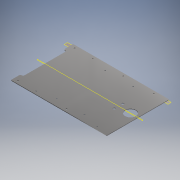
# Autodesk Inventor part: Back
Saved by Autodesk Inventor 2018 (Build 220112000, 112)
## iProperties
Created: 2017-11-12
Part Number: Back
Material: Edelstahl
Document SubType Name: Blech
Density: 8 g/cm^3
Sheet Metal Rule: Standard_mm
Appearance: Halbpoliert
Autodesk Inventor part; units mm, degrees
ref_plane "YZ Plane" through (0, 0, 0) normal (1, 0, 0) x (0, 1, 0)
ref_plane "XZ Plane" through (0, 0, 0) normal (0, 1, 0) x (-1, 0, 0)
ref_plane "XY Plane" through (0, 0, 0) normal (0, 0, 1) x (1, 0, 0)
ref_plane "Arbeitsebene1" through (0, 0, 0) normal (0, 0, 1) x (1, 0, 0)
sketch "Skizze1" plane through (0, 0, 0) normal (0, 0, 1) x (1, 0, 0)
  circle A0 centre (70.3399, -192.2557) radius 2.15 construction
  circle A1 centre (-29.6601, -192.2557) radius 2.15 construction
  circle A2 centre (-29.6601, -17.2557) radius 2.15 construction
  circle A3 centre (70.3399, -17.2557) radius 2.15 construction
  arc A4 (-167.6601, 7.2442) -> (-169.6601, 5.2442) centre (-167.6601, 5.2442) ccw construction
  line L0 (-167.6601, 7.2442) -> (173.3399, 7.2442) construction
  arc A5 (175.3399, 5.2442) -> (173.3399, 7.2442) centre (173.3399, 5.2442) ccw construction
  line L1 (175.3399, -214.7557) -> (175.3399, 5.2442) construction
  arc A6 (173.3399, -216.7557) -> (175.3399, -214.7557) centre (173.3399, -214.7557) ccw construction
  line L2 (-167.6601, -216.7557) -> (173.3399, -216.7557) construction
  arc A7 (-169.6601, -214.7557) -> (-167.6601, -216.7557) centre (-167.6601, -214.7557) ccw construction
  line L3 (-169.6601, -188.2557) -> (-169.6601, -214.7557) construction
  arc A8 (-167.6601, -186.2557) -> (-169.6601, -188.2557) centre (-167.6601, -188.2557) ccw construction
  line L4 (105.3399, -186.2557) -> (-167.6601, -186.2557) construction
  arc A9 (105.3399, -186.2557) -> (115.3399, -176.2557) centre (105.3399, -176.2557) ccw construction
  line L5 (115.3399, -33.2557) -> (115.3399, -176.2557) construction
  arc A10 (115.3399, -33.2557) -> (105.3399, -23.2557) centre (105.3399, -33.2557) ccw construction
  line L6 (-167.6601, -23.2557) -> (105.3399, -23.2557) construction
  arc A11 (-169.6601, -21.2557) -> (-167.6601, -23.2557) centre (-167.6601, -21.2557) ccw construction
  line L7 (-169.6601, 5.2442) -> (-169.6601, -21.2557) construction
  line L8 (175.3399, 7.2442) -> (-169.6601, 7.2442)
  line L9 (-169.6601, 7.2442) -> (-169.6601, -216.7557)
  line L10 (-169.6601, -216.7557) -> (175.3399, -216.7557)
  line L11 (175.3399, -216.7557) -> (175.3399, 7.2442)
  circle A12 centre (-29.6601, -17.2557) radius 2.15
  circle A13 centre (-29.6601, -192.2557) radius 2.15
  circle A14 centre (70.3399, -192.2557) radius 2.15
  circle A15 centre (70.3399, -17.2557) radius 2.15
  circle A16 centre (20.3399, -2.7558) radius 2.15
  circle A17 centre (-89.6601, -206.7557) radius 2.15
  circle A18 centre (130.3399, -206.7557) radius 2.15
  circle A19 centre (20.3399, -206.7557) radius 2.15
  circle A20 centre (-89.6601, -2.7558) radius 2.15
  circle A21 centre (130.3399, -2.7558) radius 2.15
  point P0 (0, 0)
  dimension "d0" = 0
  dimension "d1" = 345
  dimension "d2" = 193.4999
  dimension "d3" = 30.4999
  measures "d0" distance between parallel lines of L1 L11
  measures "d1" distance between parallel lines of L1 L9
  measures "d2" distance between parallel lines of L4 L8
  measures "d3" distance between parallel lines of L4 L10
extrude "Grobblech1" add sketch "Skizze1" along normal blind 2 contours L11 L10 L9 L8 | A16 | A17 | A18 | A19 | A20 | A21
fillet "Eckenrundung1" radius 2 4 edges at (-169.6601, -216.7557, 1) (175.3399, -216.7557, 1) (175.3399, 7.2442, 1) (-169.6601, 7.2442, 1)
sketch "Skizze2" plane through (0, 0, 2) normal (0, 0, 1) x (1, 0, 0)
  arc A0 (-167.6601, 7.2442) -> (-169.6601, 5.2442) centre (-167.6601, 5.2442) ccw projected
  line L0 (-169.6601, -214.7557) -> (-169.6601, 5.2442) projected
  arc A1 (-169.6601, -214.7557) -> (-167.6601, -216.7557) centre (-167.6601, -214.7557) ccw projected
  line L1 (173.3399, -216.7557) -> (-167.6601, -216.7557) projected
  arc A2 (173.3399, -216.7557) -> (175.3399, -214.7557) centre (173.3399, -214.7557) ccw projected
  line L2 (175.3399, 5.2442) -> (175.3399, -214.7557) projected
  arc A3 (175.3399, 5.2442) -> (173.3399, 7.2442) centre (173.3399, 5.2442) ccw projected
  line L3 (-167.6601, 7.2442) -> (173.3399, 7.2442) projected
  circle A4 centre (70.3399, -17.2557) radius 2.15 projected
  circle A5 centre (70.3399, -192.2557) radius 2.15 projected
  circle A6 centre (-29.6601, -192.2557) radius 2.15 projected
  circle A7 centre (-29.6601, -17.2557) radius 2.15 projected
  line L4 (-169.6601, -214.7557) -> (-169.6601, 5.2442) projected
  line L5 (-164.6601, -182.7557) -> (-164.6601, -182.7557)
  line L6 (-164.6601, -26.7558) -> (-164.6601, -26.7558)
  line L7 (-159.6601, -31.7558) -> (-159.6601, -177.7557)
  line L8 (-169.6601, -187.7557) -> (-169.6601, -214.7557)
  line L9 (-169.6601, -21.7558) -> (-169.6601, 5.2442)
  arc A8 (-169.6601, -21.7558) -> (-164.6601, -26.7558) centre (-164.6601, -21.7558) ccw
  arc A9 (-159.6601, -31.7558) -> (-164.6601, -26.7558) centre (-164.6601, -31.7558) ccw
  arc A10 (-164.6601, -182.7557) -> (-159.6601, -177.7557) centre (-164.6601, -177.7557) ccw
  arc A11 (-164.6601, -182.7557) -> (-169.6601, -187.7557) centre (-164.6601, -187.7557) ccw
  line L10 (-169.6601, -21.7558) -> (-169.6601, -187.7557)
  point P0 (0, 0)
  point P1 (-169.6601, -182.7557)
  point P2 (-159.6601, -182.7557)
  point P3 (-169.6601, -26.7558)
  point P4 (-159.6601, -26.7558)
  dimension "d6" = 10
  dimension "d7" = 34
  dimension "d8" = 10
  dimension "d9" = 34
  dimension "d10" = 5
  constraints: 12 end point, 10 point on line, 10 tangent, 8 point on circle, 4 centre point, 3 equal radius, 2 collinear, 1 horizontal, 1 perpendicular
  measures "d6" distance of point (-169.66, -182.756) point (-159.66, -182.756)
  measures "d7" distance between parallel lines of L1 L5
  measures "d8" distance of point (-169.66, -26.756) point (-159.66, -26.756)
  measures "d9" distance between parallel lines of L3 L6
  measures "d10" radius of A8
extrude "Extrusion1" cut sketch "Skizze2" against normal through all contours A8 A9 L7 A10 A11 L0
sketch "Skizze3" plane through (0, 0, 2) normal (0, 0, 1) x (1, 0, 0)
  circle A0 centre (148.5119, -104.7557) radius 16.25 projected
  circle A1 centre (148.5119, -104.7557) radius 19.25
  point P0 (0, 0)
  dimension "d27" = 3
  constraints: 1 centre point
  measures "d27" radial gap between concentric circles of A0 A1
extrude "Extrusion2" cut sketch "Skizze3" against normal through all contours A0 | A1
sketch "Skizze4" plane through (0, 0, 2) normal (0, 0, 1) x (1, 0, 0)
  line L0 (115.3399, -201.7557) -> (115.3399, -7.7558) construction
  line L1 (244.3399, -104.7557) -> (-238.6601, -104.7557) construction
  circle A0 centre (105.3399, -119.7557) radius 4
  circle A1 centre (105.3399, -89.7557) radius 4
  point P0 (0, 0)
  dimension "d15" = 8
  dimension "d16" = 8
  dimension "d17" = 15
  dimension "d18" = 10
  dimension "d19" = 10
  dimension "d20" = 15
  constraints: 2 centre point, 2 end point, 1 horizontal, 2 other
  measures "d15" diameter of A0
  measures "d16" diameter of A1
  measures "d17" distance from line of L1 A1.centre
  measures "d18" distance from line of L0 A1.centre
  measures "d19" distance from line of L0 A0.centre
  measures "d20" distance from line of L1 A0.centre
extrude "Extrusion3" cut sketch "Skizze4" against normal through all
sketch "Skizze5" plane through (0, 0, 2) normal (0, 0, 1) x (1, 0, 0)
  circle A0 centre (130.3399, -2.7558) radius 2.15 projected
  circle A1 centre (20.3399, -2.7558) radius 2.15 projected
  circle A2 centre (-89.6601, -2.7558) radius 2.15 projected
  circle A3 centre (-89.6601, -206.7557) radius 2.15 projected
  circle A4 centre (20.3399, -206.7557) radius 2.15 projected
  circle A5 centre (130.3399, -206.7557) radius 2.15 projected
  point P0 (0, 0)
extrude "Extrusion4" cut sketch "Skizze5" against normal through all
ref_plane "Arbeitsebene2" through (-167.6601, -104.7557, 0) normal (0, -1, 0) x (1, 0, 0)
sketch "Skizze6" plane through (0, 0, 0) normal (0, 0, -1) x (-1, 0, 0)
  circle A0 centre (154.6601, -2.7558) radius 2.15
  circle A1 centre (154.6601, -206.7557) radius 2.15
  point P0 (0, 0)
  constraints: 2 centre point, 4 other
extrude "Extrusion5" cut sketch "Skizze6" against normal through all
equation "\"d8\" = d6"
equation "\"d9\" = d7"
equation "\"d19\" = d18"
equation "\"d20\" = d17"
equation "\"d4\" = Stärke"
equation "\"Biegeradius\" = Stärke"
equation "\"BreiteBiegungsfreistellung\" = Stärke"
equation "\"TiefeBiegungsfreistellung\" = 0.5 * Stärke"
equation "\"GrößeEckenfreistellung\" = 4 * Stärke"
equation "\"MinimalRest\" = 2 * Stärke"
equation "\"Übergangsradius\" = Biegeradius"
equation "\"JacobiRadiusGröße\" = Biegeradius"
equation "\"Abstandsgröße\" = Stärke"
equation "\"Stärke\" = 2"
